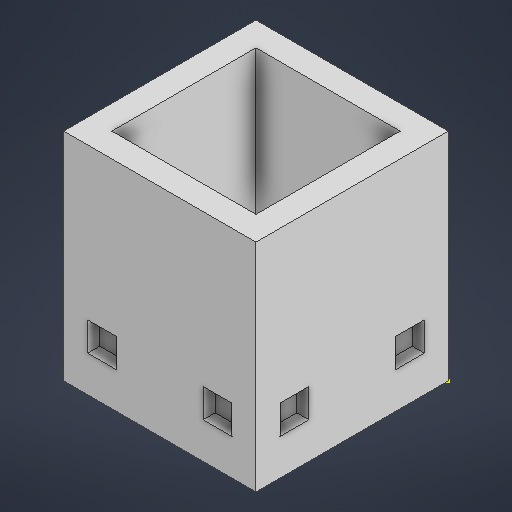
# Autodesk Inventor part: Box
Saved by Autodesk Inventor 2026 (Build 300175000, 175)
## iProperties
Created: 2025-07-03
Part Number: Box
Material: Generic
Document SubType Name: Modeling
Designer: jsmal
Density: 1 g/cm^3
Appearance: Default
Author: jsmal
Autodesk Inventor part; units mm, degrees
ref_plane "YZ Plane" through (0, 0, 0) normal (1, 0, 0) x (0, 1, 0)
ref_plane "XZ Plane" through (0, 0, 0) normal (0, 1, 0) x (-1, 0, 0)
ref_plane "XY Plane" through (0, 0, 0) normal (0, 0, 1) x (1, 0, 0)
sketch "Sketch1" plane through (0, 0, 0) normal (0, 1, 0) x (-1, 0, 0)
  line L0 (0, 0) -> (80, 0)
  line L1 (80, 0) -> (80, -80)
  line L2 (80, -80) -> (0, -80)
  line L3 (0, -80) -> (0, 0)
  dimension "d0" = 80
  dimension "d1" = 80
  constraints: 8 end point, 2 parallel, 1 horizontal, 1 perpendicular
  measures "d0" distance of L1.end L2.end
  measures "d1" distance of L0.end L1.end
extrude "Extrusion1" add sketch "Sketch1" along normal blind 10
sketch "Sketch2" plane through (0, 10, 0) normal (0, 1, 0) x (1, 0, 0)
  line L0 (-80, 0) -> (0, 0) projected
  line L1 (0, 0) -> (-80, 0)
  line L2 (-80, 0) -> (-80, 10)
  line L3 (-80, 10) -> (0, 10)
  line L4 (0, 10) -> (0, 0)
  line L5 (0, 80) -> (-80, 80) projected
  line L6 (-80, 0) -> (-70, 0)
  line L7 (-70, 0) -> (-70, 80)
  line L8 (-70, 80) -> (-80, 80)
  line L9 (-80, 80) -> (-80, 0)
  line L10 (-80, 80) -> (0, 80)
  line L11 (0, 80) -> (0, 70)
  line L12 (0, 70) -> (-80, 70)
  line L13 (-80, 70) -> (-80, 80)
  line L14 (0, 80) -> (-10, 80)
  line L15 (-10, 80) -> (-10, 0)
  line L16 (-10, 0) -> (0, 0)
  line L17 (0, 0) -> (0, 80)
  point P0 (-70, 10)
  point P1 (-70, 70)
  point P2 (-10, 70)
  point P3 (-10, 10)
  dimension "d4" = 10
  dimension "d5" = 10
  dimension "d6" = 10
  dimension "d7" = 10
  dimension "d8" = 80
  dimension "d9" = 0
  constraints: 32 end point, 8 parallel, 4 horizontal, 4 perpendicular, 3 point on line
  measures "d4" distance of L1.end L2.end
  measures "d5" distance of L8.end L7.end
  measures "d6" distance of L10.end L11.end
  measures "d7" distance of L16.end L15.end
  measures "d8" distance of L15.end L14.end
  measures "d9" distance between parallel lines of L5 L14
extrude "Extrusion2" add sketch "Sketch2" along normal blind 80 contours L2 L3 L7 L0 | L7 L3 L15 L0 | L9 L12 L7 L3 | L15 L3 L4 L0 | L9 L5 L7 L12 | L15 L12 L17 L3 | L7 L5 L15 L12 | L15 L5 L11 L12
sketch "Sketch3" plane through (-80, 0, 0) normal (0, 0, 1) x (1, 0, 0)
  line L0 (10, 27) -> (22, 27)
  line L1 (22, 27) -> (22, 15)
  line L2 (22, 15) -> (10, 15)
  line L3 (10, 15) -> (10, 27)
  line L4 (0, 0) -> (0, 90) projected
  line L5 (0, 0) -> (80, 0) projected
  line L6 (58, 27) -> (70, 27)
  line L7 (70, 27) -> (70, 15)
  line L8 (70, 15) -> (58, 15)
  line L9 (58, 15) -> (58, 27)
  line L10 (80, 0) -> (80, 90) projected
  dimension "d12" = 12
  dimension "d13" = 12
  dimension "d14" = 10
  dimension "d15" = 15
  dimension "d16" = 12
  dimension "d17" = 12
  dimension "d18" = 10
  dimension "d19" = 15
  constraints: 16 end point, 4 parallel, 2 horizontal, 2 perpendicular
  measures "d12" distance of L1.end L2.end
  measures "d13" distance of L0.end L1.end
  measures "d14" distance between parallel lines of L4 L3
  measures "d15" distance between parallel lines of L5 L2
  measures "d16" distance of L7.end L8.end
  measures "d17" distance of L6.end L7.end
  measures "d18" distance between parallel lines of L10 L7
  measures "d19" distance between parallel lines of L5 L8
sketch "Sketch4" plane through (0, 0, 0) normal (1, 0, 0) x (0, 0, -1)
  line L0 (10, 27) -> (22, 27)
  line L1 (22, 27) -> (22, 15)
  line L2 (22, 15) -> (10, 15)
  line L3 (10, 15) -> (10, 27)
  line L4 (0, 0) -> (0, 90) projected
  line L5 (0, 0) -> (80, 0) projected
  line L6 (58, 27) -> (70, 27)
  line L7 (70, 27) -> (70, 15)
  line L8 (70, 15) -> (58, 15)
  line L9 (58, 15) -> (58, 27)
  line L10 (80, 0) -> (80, 90) projected
  point P0 (16, 15)
  dimension "d20" = 12
  dimension "d21" = 12
  dimension "d22" = 10
  dimension "d23" = 15
  dimension "d24" = 12
  dimension "d25" = 12
  dimension "d26" = 10
  dimension "d27" = 15
  constraints: 16 end point, 4 parallel, 2 horizontal, 2 perpendicular, 1 midpoint
  measures "d20" distance of L1.end L2.end
  measures "d21" distance of L0.end L1.end
  measures "d22" distance between parallel lines of L4 L3
  measures "d23" distance from line of L5 point (16, 15)
  measures "d24" distance of L7.end L8.end
  measures "d25" distance of L6.end L7.end
  measures "d26" distance between parallel lines of L10 L7
  measures "d27" distance between parallel lines of L5 L8
sketch "Sketch5" plane through (0, 0, -80) normal (0, 0, -1) x (-1, 0, 0)
  line L0 (10, 27) -> (22, 27)
  line L1 (22, 27) -> (22, 15)
  line L2 (22, 15) -> (10, 15)
  line L3 (10, 15) -> (10, 27)
  line L4 (0, 0) -> (0, 90) projected
  line L5 (0, 0) -> (80, 0) projected
  line L6 (58, 27) -> (70, 27)
  line L7 (70, 27) -> (70, 15)
  line L8 (70, 15) -> (58, 15)
  line L9 (58, 15) -> (58, 27)
  line L10 (80, 0) -> (80, 90) projected
  dimension "d28" = 12
  dimension "d29" = 12
  dimension "d30" = 10
  dimension "d31" = 15
  dimension "d32" = 12
  dimension "d33" = 12
  dimension "d34" = 10
  dimension "d35" = 15
  constraints: 16 end point, 4 parallel, 2 horizontal, 2 perpendicular
  measures "d28" distance of L1.end L2.end
  measures "d29" distance of L0.end L1.end
  measures "d30" distance between parallel lines of L4 L3
  measures "d31" distance between parallel lines of L5 L2
  measures "d32" distance of L7.end L8.end
  measures "d33" distance of L6.end L7.end
  measures "d34" distance between parallel lines of L10 L7
  measures "d35" distance between parallel lines of L5 L8
sketch "Sketch6" plane through (0, 0, -80) normal (0, 0, -1) x (-1, 0, 0)
  point P0 (0, 0)
sketch "Sketch7" plane through (-80, 0, -80) normal (-1, 0, 0) x (0, 0, 1)
  line L0 (10, 27) -> (22, 27)
  line L1 (22, 27) -> (22, 15)
  line L2 (22, 15) -> (10, 15)
  line L3 (10, 15) -> (10, 27)
  line L4 (0, 0) -> (0, 90) projected
  line L5 (0, 0) -> (80, 0) projected
  line L6 (58, 27) -> (70, 27)
  line L7 (70, 27) -> (70, 15)
  line L8 (70, 15) -> (58, 15)
  line L9 (58, 15) -> (58, 27)
  line L10 (80, 0) -> (80, 90) projected
  point P0 (16, 15)
  dimension "d36" = 12
  dimension "d37" = 12
  dimension "d38" = 10
  dimension "d39" = 15
  dimension "d40" = 12
  dimension "d41" = 12
  dimension "d42" = 10
  dimension "d43" = 15
  constraints: 16 end point, 4 parallel, 2 horizontal, 2 perpendicular, 1 midpoint
  measures "d36" distance of L1.end L2.end
  measures "d37" distance of L0.end L1.end
  measures "d38" distance between parallel lines of L4 L3
  measures "d39" distance from line of L5 point (16, 15)
  measures "d40" distance of L7.end L8.end
  measures "d41" distance of L6.end L7.end
  measures "d42" distance between parallel lines of L10 L7
  measures "d43" distance between parallel lines of L5 L8
extrude "Extrusion3" cut sketch "Sketch7" against normal blind 5
extrude "Extrusion4" cut sketch "Sketch4" against normal blind 5
extrude "Extrusion5" cut sketch "Sketch3" against normal blind 5
extrude "Extrusion6" cut sketch "Sketch5" against normal blind 5
body "Solid1"
